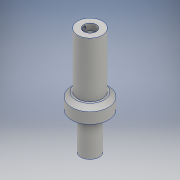
# Autodesk Inventor part: koncowka
Saved by Autodesk Inventor 2017 (Build 210142000, 142)
## iProperties
Created: 2017-03-22
Part Number: koncowka
Material: Aluminium 6061
Document SubType Name: Modeling
Designer: Damian
Density: 2.7 g/cm^3
Appearance: Aluminium — płaski
Mass: 77.3226 g
Surface Area: 67.3428 cm^2
Volume: 28.638 cm^3
Author: Damian
Autodesk Inventor part; units mm, degrees
ref_plane "YZ Plane" through (0, 0, 0) normal (1, 0, 0) x (0, 1, 0)
ref_plane "XZ Plane" through (0, 0, 0) normal (0, 1, 0) x (-1, 0, 0)
ref_plane "XY Plane" through (0, 0, 0) normal (0, 0, 1) x (1, 0, 0)
sketch "Szkic1" plane through (0, 0, 0) normal (0, 0, 1) x (1, 0, 0)
  circle A0 centre (0, 0) radius 15
  dimension "d0" = 30
  constraints: 1 centre point, 1 coincident
  measures "d0" diameter of A0
extrude "Wyciągnięcie proste1" add sketch "Szkic1" along normal blind 35 and the other way blind 37.5
sketch "Szkic3" plane through (0, 0, 35) normal (0, 0, 1) x (1, 0, 0)
  circle A0 centre (0, 0) radius 10
  circle A1 centre (0, 0) radius 15
  dimension "d4" = 20
  dimension "d5" = 30
  constraints: 3 coincident, 2 centre point
  measures "d4" diameter of A0
  measures "d5" diameter of A1
extrude "Wyciągnięcie proste2" cut sketch "Szkic3" against normal blind 30
chamfer "Faza1" distance 3.5 angle 45 1 edges at (-15, 0, 5)
sketch "Szkic4" plane through (0, 0, -37.5) normal (0, 0, -1) x (-1, 0, 0)
  circle A0 centre (0, 0) radius 7.5
  circle A1 centre (0, 0) radius 15
  dimension "d11" = 15
  dimension "d12" = 30
  constraints: 3 coincident, 2 centre point
  measures "d11" diameter of A0
  measures "d12" diameter of A1
extrude "Wyciągnięcie proste3" cut sketch "Szkic4" against normal blind 30
sketch "Szkic8" plane through (0, 0, 35) normal (0, 0, 1) x (1, 0, 0)
  circle A0 centre (0, 0) radius 10
  dimension "d33" = 20
  constraints: 1 centre point, 1 coincident
  measures "d33" diameter of A0
extrude "Wyciągnięcie proste7" add sketch "Szkic8" along normal blind 15
sketch "Szkic9" plane through (0, 0, 50) normal (0, 0, 1) x (1, 0, 0)
  circle A0 centre (0, 0) radius 5.05
  dimension "d36" = 10.1
  constraints: 1 centre point, 1 coincident
  measures "d36" diameter of A0
extrude "Wyciągnięcie proste8" cut sketch "Szkic9" against normal blind 5.5
sketch "Szkic10" plane through (0, 0, 0) normal (1, 0, 0) x (0, 1, 0)
  circle A0 centre (0, 47.5) radius 1.5
  line L0 (-5.05, 50) -> (5.05, 50) projected
  point P0 (0, 0)
  dimension "d39" = 3
  dimension "d42" = 2.5
  constraints: 1 centre point
  measures "d39" diameter of A0
  measures "d42" distance from line of L0 A0.centre
extrude "Wyciągnięcie proste9" cut sketch "Szkic10" against normal blind 25
thread "Gwint4" size "M3x0.5" class "6H" standard "ANSI Metric M Profile" full length
sketch "Szkic11" plane through (0, 0, 0) normal (1, 0, 0) x (0, 1, 0)
  circle A0 centre (0, -22.5) radius 1.5
  point P0 (0, 0)
  dimension "d45" = 3
  constraints: 1 centre point
  measures "d45" diameter of A0
extrude "Wyciągnięcie proste10" cut sketch "Szkic11" against normal blind 20
thread "Gwint5" size "M3x0.5" class "6H" standard "ANSI Metric M Profile" full length
